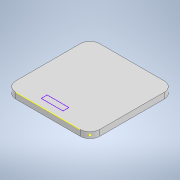
# Autodesk Inventor part: NewBase
Saved by Autodesk Inventor 2020.1 (Build 241239000, 239)
## iProperties
Created: 2020-02-26
Part Number: NewBase
Material: Generic
Document SubType Name: Modeling
Designer: super
Density: 1 g/cm^3
Appearance: Default
Author: super
Autodesk Inventor part; units mm, degrees
ref_plane "YZ Plane" through (0, 0, 0) normal (1, 0, 0) x (0, 1, 0)
ref_plane "XZ Plane" through (0, 0, 0) normal (0, 1, 0) x (-1, 0, 0)
ref_plane "XY Plane" through (0, 0, 0) normal (0, 0, 1) x (1, 0, 0)
sketch "Sketch1" plane through (0, 0, 0) normal (0, 1, 0) x (-1, 0, 0)
  line L0 (0, 0) -> (85, 0)
  line L1 (85, 0) -> (85, -85)
  line L2 (85, -85) -> (0, -85)
  line L3 (0, -85) -> (0, 0)
  dimension "d0" = 85
  dimension "d1" = 85
  constraints: 8 end point, 2 parallel, 1 horizontal, 1 perpendicular
  measures "d0" distance of L1.end L2.end
  measures "d1" distance of L0.end L1.end
extrude "Extrusion1" add sketch "Sketch1" along normal blind 6
fillet "Fillet1" radius 10 4 edges at (-85, 3, 0) (0, 3, 0) (0, 3, -85) (-85, 3, -85)
sketch "Sketch2" plane through (0, 6, 0) normal (0, 1, 0) x (1, 0, 0)
  line L0 (-75, 0) -> (-10, 0) projected
  line L1 (-57, 7.5) -> (-35, 7.5)
  line L2 (-35, 7.5) -> (-35, 12.5)
  line L3 (-35, 12.5) -> (-35, 13.5)
  line L4 (-35, 13.5) -> (-57, 13.5)
  line L5 (-57, 13.5) -> (-57, 7.5)
  point P0 (0, 0)
  constraints: 10 end point, 3 perpendicular, 1 point on line
body "Solid1"
